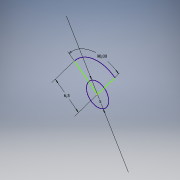
# Autodesk Inventor part: encoder_pole
Saved by Autodesk Inventor 2019.4 (Build 234330000, 330)
## iProperties
Created: 2020-06-20
Part Number: encoder_pole
Material: Generic
Document SubType Name: Modeling
Designer: Jorge
Density: 1 g/cm^3
Appearance: Default
Author: Jorge
Autodesk Inventor part; units mm, degrees
ref_plane "YZ Plane" through (0, 0, 0) normal (1, 0, 0) x (0, 1, 0)
ref_plane "XZ Plane" through (0, 0, 0) normal (0, 1, 0) x (-1, 0, 0)
ref_plane "XY Plane" through (0, 0, 0) normal (0, 0, 1) x (1, 0, 0)
sketch "Sketch1" plane through (0, 0, 0) normal (0, 0, 1) x (1, 0, 0)
  arc A0 (1.6837, 1.848) -> (-1.848, 1.6837) centre (0, 0) ccw
  line L0 (0, 0) -> (-1.848, 1.6837) construction
  arc A1 (4.3777, 4.8047) -> (-4.8047, 4.3777) centre (0, 0) ccw
  line L1 (0, 0) -> (1.6837, 1.848) construction
  arc A2 (-1.848, 1.6837) -> (1.6837, 1.848) centre (0, 0) ccw construction
  line L2 (1.6837, 1.848) -> (4.3777, 4.8047)
  line L3 (-1.848, 1.6837) -> (-4.8047, 4.3777)
  dimension "d0" = 5
  dimension "d2" = 6.5
  constraints: 8 end point, 6 point on circle, 3 centre point, 2 coincident, 1 perpendicular
  measures "d0" diameter of A0
  measures "d2" distance of L0.start L3.end
extrude "Extrusion1" add sketch "Sketch1" along normal blind 3.5
body "Solid1"
